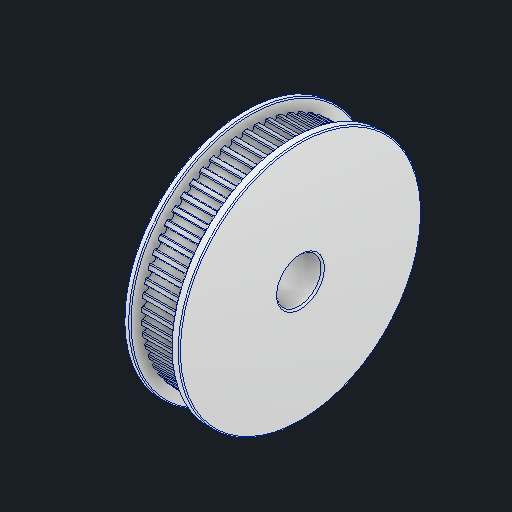
# Autodesk Inventor part: GT2Pulley_z60
Saved by Autodesk Inventor 2025.2 (Build 292293000, 293)
## iProperties
Created: 2025-05-15
Part Number: GT2Pulley_z60
Material: Stainless Steel
Document SubType Name: Modeling
Designer: Tiago
Density: 8 g/cm^3
Appearance: Aluminum - Flat
Mass: 116.469 g
Surface Area: 62.5344 cm^2
Volume: 14.5586 cm^3
Author: Tiago
Autodesk Inventor part; units mm, degrees
ref_plane "YZ Plane" through (0, 0, 0) normal (1, 0, 0) x (0, 1, 0)
sketch "Sketch1" plane through (0, 0, 0) normal (0, 0, 1) x (1, 0, 0)
  line L0 (0, 4) -> (0, 21.8001)
  line L1 (0, 21.8001) -> (7.1, 21.8001)
  line L2 (7.1, 21.8001) -> (7.1, 18.8426)
  line L3 (7.1, 18.8426) -> (14.5, 18.8426)
  line L4 (14.5, 18.8426) -> (14.5, 21.8001)
  line L5 (14.5, 21.8001) -> (16, 21.8001)
  line L6 (16, 21.8001) -> (16, 4)
  line L7 (16, 0) -> (0, 0)
  line L8 (0, 4) -> (16, 4)
  line L9 (0, 12.5) -> (6, 12.5)
  line L10 (6, 12.5) -> (6, 21.8001)
  dimension "L" = 16
  dimension "d1" = 7.1
  dimension "DE" = 43.6002
  dimension "d3" = 37.6852
  dimension "d4" = 7.4
  dimension "d5" = 43.6002
  dimension "Bore" = 8
  dimension "d33" = 25
  dimension "d34" = 6
  constraints: 22 end point, 8 perpendicular, 2 horizontal, 2 point on line, 2 vertical alignment, 1 vertical
  measures "L" distance of L7.start L7.end
  measures "d1" distance between parallel lines of L0 L2
  measures "DE" diameter of L1 L7
  measures "d3" diameter of L3 L7
  measures "d4" distance between parallel lines of L4 L2
  measures "d5" diameter of L5 L7
  measures "Bore" diameter of L8 L7
  measures "d33" diameter of L9 L7
  measures "d34" distance of L9.start L9.end
revolve "Revolution1" add sketch "Sketch1" angle 360 about axis through (16, 0, 0) along (-1, 0, 0) contours L0 L9 L10 L1 L2 L3 L4 L5 L6 L8
sketch "Sketch3" plane through (7.1, 0, 0) normal (1, 0, 0) x (0, 0, -1)
  line L0 (0, 0) -> (0, 8.9731) construction
  line L1 (0, 0) -> (0.4945, 9.4347) construction
  line L2 (0, 0) -> (0.7013, 9.5505) construction
  line L3 (0, 0) -> (0.9738, 9.2647) construction
  circle A0 centre (0, 0) radius 18.8426
  circle A1 centre (0, 0) radius 19.3976 construction
  arc A2 (1.5017, 19.4687) -> (1.37, 19.6663) centre (1.3596, 19.5167) ccw
  arc A3 (1.5017, 19.4687) -> (1.9696, 18.7394) centre (2.0276, 19.2913) ccw
  arc A4 (0.6932, 19.7018) -> (0.5416, 19.519) centre (0.6879, 19.5519) ccw
  arc A5 (0, 18.8426) -> (0.5416, 19.519) centre (0, 19.3976) ccw
  circle A6 centre (0, 0.0002) radius 19.0986 construction
  arc A7 (1.37, 19.6663) -> (0.6932, 19.7018) centre (0, 0) ccw
  point P0 (0, 18.8426)
  dimension "di" = 37.6852
  dimension "d12" = 0.555
  dimension "d8" = 3
  dimension "ANGLEP" = 6
  dimension "d10" = 1.2
  dimension "d16" = 0.3
  dimension "d17" = 0.555
  dimension "d18" = 0.15
  dimension "PD" = 38.1972
  constraints: 10 point on circle, 8 end point, 6 centre point, 5 symmetric about line, 2 tangent, 1 coincident, 1 point on line, 1 vertical, 8 other
  measures "d8" angle of L0 L1
  measures "ANGLEP" angle of L0 L3
  measures "d10" angle of L1 L2
  measures "d16" diameter of A2
  measures "d17" radius of A3
  measures "d18" radius of A2
  measures "PD" diameter of A6
extrude "Extrusion2" add sketch "Sketch3" along normal up to surface (7.4 mm away) contours A0 A5 A4 A7 A2 A3
pattern_circular "Circular Pattern2" count 60 over 360 about axis through (-10, 0, 0) along (1, 0, 0) of "Extrusion2"
ref_plane "Work Plane1" through (3, 12.5, 0) normal (0, 1, 0) x (-1, 0, 0)
sketch "Sketch4" plane through (3, 12.5, 0) normal (0, 1, 0) x (-1, 0, 0)
  circle A0 centre (-0.5, 0) radius 1.5
  line L0 (3, -12.5) -> (3, 12.5) projected
  point P0 (3, 0)
  dimension "d35" = 3
  dimension "d36" = 3.5
  constraints: 1 centre point, 1 horizontal alignment
  measures "d35" diameter of A0
  measures "d36" distance from line of A0.centre L0
extrude "Extrusion3" cut sketch "Sketch4" against normal up to surface
ref_plane "Work Plane2" through (3, 0, 12.5) normal (0, 0, 1) x (1, 0, 0)
sketch "Sketch5" plane through (3, 0, 12.5) normal (0, 0, 1) x (1, 0, 0)
  circle A0 centre (0.5, 0) radius 1.5
  line L0 (-3, 12.5) -> (-3, -12.5) projected
  point P0 (-3, 0)
  dimension "d39" = 3
  dimension "d40" = 3.5
  constraints: 1 centre point, 1 horizontal alignment
  measures "d39" diameter of A0
  measures "d40" distance from line of L0 A0.centre
extrude "Extrusion4" cut sketch "Sketch5" against normal up to surface
fillet "Fillet1" radius 0.2 4 edges at (16, -21.8001, 0) (7.1, -21.8001, 0) (6, -21.8001, 0) (14.5, -21.8001, 0)
fillet "Fillet2" radius 0.3 7 edges at (16, -4, 0) (0, -12.5, 0) (0, -4, 0) (3.4987, 12.4097, -1.5) (3.4999, 12.4097, 1.5) (3.5003, 1.5, 12.4097) (3.3637, -1.4938, 12.4104)
equation "\"d3\" = di"
equation "\"d5\" = DE"
equation "\"d8\" = 0.5 * ANGLEP"
equation "\"d10\" = 0.2 * ANGLEP"
equation "\"PD\" = 0.63662 * zz"
equation "\"zz\" = 60"
body "Solid1"
